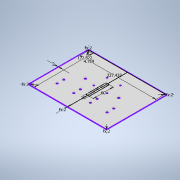
# Autodesk Inventor part: EboxBottom
Saved by Autodesk Inventor 2021 (Build 250183000, 183)
## iProperties
Created: 2022-01-03
Part Number: EboxBottom
Material: Generic
Document SubType Name: Modeling
Designer: Jorian Brusind
Density: 1 g/cm^3
Appearance: Default
Author: Jorian Brusind
Autodesk Inventor part; units mm, degrees
ref_plane "YZ Plane" through (0, 0, 0) normal (1, 0, 0) x (0, 1, 0)
ref_plane "XZ Plane" through (0, 0, 0) normal (0, 1, 0) x (-1, 0, 0)
ref_plane "XY Plane" through (0, 0, 0) normal (0, 0, 1) x (1, 0, 0)
sketch "Sketch1" plane through (0, 0, 0) normal (0, 1, 0) x (-1, 0, 0)
  line L0 (232.1908, -176.5808) -> (232.1908, -3.7592)
  arc A0 (232.1908, -3.7592) -> (227.4316, 1) centre (227.4316, -3.7592) ccw
  line L1 (227.4316, 1) -> (0, 1)
  arc A1 (0, 1) -> (-4.7592, -3.7592) centre (0, -3.7592) ccw
  arc A2 (-4.7592, -176.5808) -> (0, -181.34) centre (0, -176.5808) ccw
  arc A3 (227.4316, -181.34) -> (232.1908, -176.5808) centre (227.4316, -176.5808) ccw
  circle A4 centre (130, -135) radius 2
  circle A5 centre (130, -95) radius 2
  circle A6 centre (90, -135) radius 2
  circle A7 centre (90, -95) radius 2
  circle A8 centre (160.0797, -100) radius 2.75
  circle A9 centre (60.0797, -100) radius 2.75
  circle A10 centre (90, -45) radius 2.5
  circle A11 centre (190, -45) radius 2.5
  circle A12 centre (190, -65) radius 2.5
  circle A13 centre (90, -65) radius 2.5
  circle A14 centre (140, -45) radius 2.5
  circle A15 centre (40, -45) radius 2.5
  circle A16 centre (140, -65) radius 2.5
  circle A17 centre (40, -65) radius 2.5
  line L2 (230.1908, -176.5808) -> (230.1908, -3.7592)
  arc A18 (230.1908, -3.7592) -> (227.4316, -1) centre (227.4316, -3.7592) ccw
  line L3 (227.4316, -1) -> (0, -1)
  arc A19 (0, -1) -> (-2.7592, -3.7592) centre (0, -3.7592) ccw
  arc A20 (-2.7592, -176.5808) -> (0, -179.34) centre (0, -176.5808) ccw
  arc A21 (227.4316, -179.34) -> (230.1908, -176.5808) centre (227.4316, -176.5808) ccw
  line L4 (-4.7592, -3.7592) -> (-4.7592, -176.5808)
  line L5 (-2.7592, -3.7592) -> (-2.7592, -176.5808)
  line L6 (0, -179.34) -> (227.4316, -179.34)
  line L7 (227.4316, -181.34) -> (0, -181.34)
  point P0 (0, 0)
  point P1 (230.1908, -3.7592)
  point P2 (0, -1)
  dimension "d0" = 2
  dimension "d1" = 2
  dimension "d2" = 2
  dimension "d3" = 2
  dimension "d5" = 2
  dimension "d7" = 2
  dimension "d8" = 227.4316
  dimension "d9" = 172.8216
  dimension "d10" = 4.7592
  constraints: 22 centre point, 16 end point, 16 point on circle, 4 parallel, 1 horizontal, 1 tangent, 1 vertical
  measures "d0" distance between parallel lines of L0 L2
  measures "d1" radial gap between concentric circles of A0 A18
  measures "d2" distance between parallel lines of L1 L3
  measures "d3" radial gap between concentric circles of A1 A19
  measures "d5" radial gap between concentric circles of A2 A20
  measures "d7" radial gap between concentric circles of A3 A21
  measures "d8" distance of L7.start L7.end
  measures "d9" distance of L0.start L0.end
  measures "d10" radius of A3
extrude "Extrusion1" add sketch "Sketch1" along normal blind 3 contours A21 L6 A20 L5 A19 L3 A18 L2
sketch "Sketch2" plane through (0, 3, 0) normal (0, 1, 0) x (1, 0, 0)
  line L0 (-232.1908, 176.5808) -> (-232.1908, 3.7592)
  arc A0 (-232.1908, 3.7592) -> (-227.4316, -1) centre (-227.4316, 3.7592) ccw
  line L1 (-227.4316, -1) -> (0, -1)
  arc A1 (0, -1) -> (4.7592, 3.7592) centre (0, 3.7592) ccw
  arc A2 (4.7592, 176.5808) -> (0, 181.34) centre (0, 176.5808) ccw
  arc A3 (-227.4316, 181.34) -> (-232.1908, 176.5808) centre (-227.4316, 176.5808) ccw
  circle A4 centre (-130, 135) radius 2
  circle A5 centre (-130, 95) radius 2
  circle A6 centre (-90, 135) radius 2
  circle A7 centre (-90, 95) radius 2
  circle A8 centre (-160.0797, 100) radius 2.75
  circle A9 centre (-60.0797, 100) radius 2.75
  circle A10 centre (-90, 45) radius 2.5
  circle A11 centre (-190, 45) radius 2.5
  circle A12 centre (-190, 65) radius 2.5
  circle A13 centre (-90, 65) radius 2.5
  circle A14 centre (-140, 45) radius 2.5
  circle A15 centre (-40, 45) radius 2.5
  circle A16 centre (-140, 65) radius 2.5
  circle A17 centre (-40, 65) radius 2.5
  line L2 (-230.1908, 176.5808) -> (-230.1908, 3.7592)
  arc A18 (-230.1908, 3.7592) -> (-227.4316, 1) centre (-227.4316, 3.7592) ccw
  line L3 (-227.4316, 1) -> (0, 1)
  arc A19 (0, 1) -> (2.7592, 3.7592) centre (0, 3.7592) ccw
  arc A20 (2.7592, 176.5808) -> (0, 179.34) centre (0, 176.5808) ccw
  arc A21 (-227.4316, 179.34) -> (-230.1908, 176.5808) centre (-227.4316, 176.5808) ccw
  line L4 (4.7592, 3.7592) -> (4.7592, 176.5808)
  line L5 (2.7592, 3.7592) -> (2.7592, 176.5808)
  line L6 (0, 179.34) -> (-227.4316, 179.34)
  line L7 (-227.4316, 181.34) -> (0, 181.34)
  line L8 (0, 179.34) -> (-227.4316, 179.34) projected
  line L9 (-113.7158, 179.34) -> (-113.7158, 1)
  line L10 (-227.4316, 1) -> (0, 1) projected
  line L11 (-118.7158, 120.17) -> (-108.7158, 120.17)
  line L12 (-108.7158, 120.17) -> (-108.7158, 60.17)
  line L13 (-108.7158, 60.17) -> (-118.7158, 60.17)
  line L14 (-118.7158, 60.17) -> (-118.7158, 120.17)
  line L15 (-118.7158, 120.17) -> (-108.7158, 60.17) construction
  line L16 (-108.7158, 120.17) -> (-118.7158, 60.17) construction
  point P0 (230.1908, -176.5808)
  point P1 (230.1908, -3.7592)
  point P2 (227.4316, -1)
  point P3 (0, -1)
  point P4 (0, 0)
  point P5 (230.1908, -176.5808)
  point P6 (230.1908, -3.7592)
  point P7 (227.4316, -1)
  point P8 (0, -1)
  point P9 (-113.7158, 90.17)
  dimension "d22" = 2
  dimension "d23" = 2
  dimension "d24" = 2
  dimension "d25" = 2
  dimension "d26" = 2
  dimension "d27" = 2
  dimension "d28" = 227.4316
  dimension "d29" = 172.8216
  dimension "d30" = 4.7592
  dimension "d31" = 10
  dimension "d32" = 60
  constraints: 30 end point, 22 centre point, 16 point on circle, 6 parallel, 5 midpoint, 1 horizontal, 1 perpendicular, 1 tangent
  measures "d22" distance between parallel lines of L0 L2
  measures "d23" radial gap between concentric circles of A0 A18
  measures "d24" distance between parallel lines of L1 L3
  measures "d25" radial gap between concentric circles of A1 A19
  measures "d26" radial gap between concentric circles of A2 A20
  measures "d27" radial gap between concentric circles of A3 A21
  measures "d28" distance of L7.start L7.end
  measures "d29" distance of L0.start L0.end
  measures "d30" radius of A3
  measures "d31" distance of L12.end L13.end
  measures "d32" distance of L11.end L12.end
equation "\"d1\" = d0"
equation "\"d2\" = d0"
equation "\"d3\" = d0"
equation "\"d5\" = d0"
equation "\"d7\" = d0"
equation "\"d23\" = d22"
equation "\"d24\" = d22"
equation "\"d25\" = d22"
equation "\"d26\" = d22"
equation "\"d27\" = d22"
body "Solid1"
